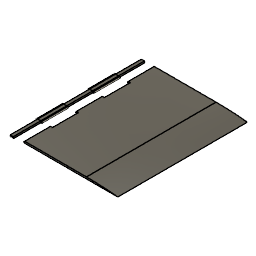
Expandable Notebook (Autodesk Fusion 360 design; units mm, degrees)
Autodesk Fusion 360 part; units mm, degrees
sketch "Sketch1" plane through (0, 0, 0) normal (0, 0, 1) x (1, 0, 0)
  line L0 (0, 0) -> (-148.5, 0)
  line L1 (-148.5, 0) -> (-148.5, 210)
  line L2 (-148.5, 210) -> (0, 210)
  line L3 (0, 210) -> (0, 0)
  line L4 (0, 0) -> (7.0711, -7.0711)
  line L5 (0, 0) -> (10, 0) construction
  line L6 (-148.5, 210) -> (-155.5711, 217.0711)
  line L7 (-148.5, 210) -> (-138.5, 210) construction
  line L8 (-155.5711, 217.0711) -> (7.0711, 217.0711)
  line L9 (7.0711, 217.0711) -> (7.0711, -7.0711)
  line L10 (7.0711, -7.0711) -> (-155.5711, -7.0711)
  line L11 (-155.5711, -7.0711) -> (-155.5711, 217.0711)
  dimension "d1" = 148.5
  dimension "d2" = 210
  dimension "d3" = 10
  dimension "d4" = 45
  dimension "d5" = 135
  dimension "d6" = 10
  constraint horizontal L0
  constraint vertical L1
  constraint horizontal L2
  constraint vertical L3
  constraint coincident L0.start L3.end
  constraint horizontal L5
  constraint horizontal L7
  constraint horizontal L8
  constraint vertical L9
  constraint horizontal L10
  constraint vertical L11
  measures "d1" distance of L0.start L0.end
  measures "d2" distance of L0.start L2.end
  measures "d3" distance of L0.start L4.end
  measures "d4" angle of L4 L5
  measures "d5" angle of L6 L7
  measures "d6" distance of L1.end L6.end
extrude "Extrude1" add sketch "Sketch1" along normal blind 3 makes body 1
sketch "Sketch2" plane through (0, 0, 3) normal (0, 0, 1) x (-1, 0, 0)
  line L0 (155.5711, 7.0711) -> (-7.0711, 7.0711)
  line L1 (-7.0711, 7.0711) -> (-7.0711, -217.0711)
  line L2 (-7.0711, -217.0711) -> (155.5711, -217.0711)
  line L3 (155.5711, -217.0711) -> (155.5711, 7.0711)
  line L4 (155.5711, 7.0711) -> (145.5711, 7.0711)
  line L5 (145.5711, 7.0711) -> (145.5711, -217.0709)
  line L6 (145.5711, -217.0709) -> (155.5711, -217.0709)
  line L7 (155.5711, -217.0709) -> (155.5711, 7.0711)
  line L8 (155.5711, -217.0711) -> (150.5711, -217.0711)
  line L9 (150.5711, -217.0711) -> (150.5711, -172.2427)
  line L10 (150.5711, -172.2427) -> (155.5711, -172.2427)
  line L11 (155.5711, -172.2427) -> (155.5711, -217.0711)
  line L12 (150.5711, -172.2427) -> (155.5711, -172.2427)
  line L13 (155.5711, -172.2427) -> (155.5711, -127.4143)
  line L14 (155.5711, -127.4143) -> (150.5711, -127.4143)
  line L15 (150.5711, -127.4143) -> (150.5711, -172.2427)
  line L16 (150.5711, -127.4143) -> (155.5711, -127.4143)
  line L17 (155.5711, -127.4143) -> (155.5711, -82.5859)
  line L18 (155.5711, -82.5859) -> (150.5711, -82.5859)
  line L19 (150.5711, -82.5859) -> (150.5711, -127.4143)
  line L20 (150.5711, -82.5859) -> (155.5711, -82.5859)
  line L21 (155.5711, -82.5859) -> (155.5711, -37.7575)
  line L22 (155.5711, -37.7575) -> (150.5711, -37.7575)
  line L23 (150.5711, -37.7575) -> (150.5711, -82.5859)
  line L24 (150.5711, -37.7575) -> (155.5711, -37.7575)
  line L25 (155.5711, -37.7575) -> (155.5711, 7.0711)
  line L26 (155.5711, 7.0711) -> (150.5711, 7.0711)
  line L27 (150.5711, 7.0711) -> (150.5711, -37.7575)
  dimension "d9" = 10
  dimension "d10" = 224.142
  dimension "d11" = 44.8284
  dimension "d12" = 44.8284
  dimension "d13" = 44.8284
  dimension "d14" = 44.8284
  constraint horizontal L4
  constraint vertical L5
  constraint horizontal L6
  constraint vertical L7
  constraint coincident L0.start L3.end
  constraint horizontal L8
  constraint vertical L9
  constraint horizontal L10
  constraint vertical L11
  constraint coincident L2.end L3.start
  constraint horizontal L12
  constraint vertical L13
  constraint horizontal L14
  constraint vertical L15
  constraint horizontal L16
  constraint vertical L17
  constraint horizontal L18
  constraint vertical L19
  constraint coincident L7 L17.end
  constraint horizontal L20
  constraint vertical L21
  constraint horizontal L22
  constraint vertical L23
  constraint coincident L7 L21.end
  constraint horizontal L24
  constraint vertical L25
  constraint horizontal L26
  constraint vertical L27
  measures "d9" distance of L0.start L4.end
  measures "d10" distance of L0.start L6.end
  measures "d11" distance of L2.end L10.end
  measures "d12" distance of L9.end L14.end
  measures "d13" distance of L14.end L18.end
  measures "d14" distance of L18.end L22.end
extrude "Extrude2" cut sketch "Sketch2" against normal blind 160 contours L3 L7 L18 L20 L21 L22 L23 L24 | L3 L7 L10 L12 L13 L14 L15 L16 bodies 1
sketch "Sketch3" plane through (0, 0, 0) normal (0, 0, 1) x (1, 0, 0)
  line L0 (-170.5711, 217.0711) -> (-176.0711, 217.0711)
  line L1 (-176.0711, 217.0711) -> (-176.0711, -9.7901)
  line L2 (-176.0711, -9.7901) -> (-170.5711, -9.7901)
  line L3 (-170.5711, -9.7901) -> (-170.5711, 217.0711)
  line L4 (-170.5711, 217.0711) -> (-170.5711, 172.2427)
  line L5 (-170.5711, 127.4143) -> (-170.5711, 82.5859)
  line L6 (-170.5711, 82.5859) -> (-170.5711, 37.7575)
  line L7 (-170.5711, 37.7575) -> (-167.5711, 37.7575)
  line L8 (-167.5711, 37.7575) -> (-167.5711, 82.5859)
  line L9 (-167.5711, 82.5859) -> (-170.5711, 82.5859)
  line L10 (-170.5711, 82.5859) -> (-170.5711, 37.7575)
  line L11 (-176.0711, 172.2427) -> (-179.0711, 172.2427)
  line L12 (-179.0711, 172.2427) -> (-179.0711, 127.4143)
  line L13 (-179.0711, 127.4143) -> (-176.0711, 127.4143)
  line L14 (-176.0711, 127.4143) -> (-176.0711, 172.2427)
  line L15 (-170.5711, 82.5859) -> (-176.0711, 82.5859)
  line L16 (-176.0711, 82.5859) -> (-176.0711, 37.7575)
  line L17 (-176.0711, 37.7575) -> (-170.5711, 37.7575)
  line L18 (-170.5711, 37.7575) -> (-170.5711, 82.5859)
  line L19 (-176.0711, 37.7575) -> (-179.0711, 37.7575)
  line L20 (-179.0711, 37.7575) -> (-179.0711, 82.5859)
  line L21 (-179.0711, 82.5859) -> (-176.0711, 82.5859)
  line L22 (-176.0711, 82.5859) -> (-176.0711, 37.7575)
  line L23 (-170.5711, 172.2427) -> (-167.5711, 172.2427)
  line L24 (-167.5711, 172.2427) -> (-167.5711, 127.4143)
  line L25 (-167.5711, 127.4143) -> (-170.5711, 127.4143)
  line L26 (-170.5711, 127.4143) -> (-170.5711, 172.2427)
  point P0 (-155.5711, 217.0711)
  point P1 (-155.5711, -7.0711)
  dimension "d17" = 15
  dimension "d19" = 5.5
  dimension "d20" = 44.8284
  dimension "d21" = 44.8284
  dimension "d22" = 44.8284
  dimension "d23" = 44.8284
  dimension "d24" = 3
  dimension "d25" = 44.8284
  dimension "d27" = 3
  dimension "d28" = 44.8284
  dimension "d29" = 3
  dimension "d30" = 3
  dimension "d31" = 44.8284
  constraint horizontal L0
  constraint vertical L1
  constraint horizontal L2
  constraint vertical L3
  constraint coincident L3 L5.start
  constraint horizontal L7
  constraint vertical L8
  constraint horizontal L9
  constraint vertical L10
  constraint horizontal L11
  constraint vertical L12
  constraint horizontal L13
  constraint vertical L14
  constraint coincident L1 L11.start
  constraint horizontal L15
  constraint vertical L16
  constraint horizontal L17
  constraint vertical L18
  constraint coincident L1 L16.end
  constraint horizontal L19
  constraint vertical L20
  constraint horizontal L21
  constraint vertical L22
  constraint horizontal L23
  constraint vertical L24
  constraint horizontal L25
  constraint vertical L26
  measures "d17" distance of P0 L0.start
  measures "d19" distance of L0.start L0.end
  measures "d20" distance of L0.start L4.end
  measures "d21" distance of L4.end L5.start
  measures "d22" distance of L5.start L5.end
  measures "d23" distance of L5.end L6.end
  measures "d24" distance of L6.end L7.end
  measures "d25" distance of L6.end L5.end
  measures "d27" distance of L11.start L11.end
  measures "d28" distance of L5.end L6.end
  measures "d29" distance of L16.end L19.end
  measures "d30" distance of L4.end L23.end
  measures "d31" distance of L4.end L5.start
extrude "Extrude3" add sketch "Sketch3" along normal blind 3 separate body makes body 2
fillet "Fillet1" radius 1.5 8 edges at (-179.0711, 60.1717, 0) (-179.0711, 60.1717, 3) (-179.0711, 149.8285, 0) (-179.0711, 149.8285, 3) (-167.5711, 60.1717, 0) (-167.5711, 60.1717, 3) (-167.5711, 149.8285, 0) (-167.5711, 149.8285, 3) on bodies 2
fillet "Fillet2" radius 1.5 6 edges at (-155.5711, 194.6569, 3) (-155.5711, 194.6569, 0) (-155.5711, 105.0001, 0) (-155.5711, 105.0001, 3) (-155.5711, 15.3432, 3) (-155.5711, 15.3432, 0) on bodies 1
sketch "Sketch4" plane through (0, 217.0711, 0) normal (0, 1, 0) x (-1, 0, 0)
  line L0 (170.5711, 0) -> (176.0711, 0)
  line L1 (176.0711, 0) -> (176.0711, 3)
  line L2 (176.0711, 3) -> (170.5711, 3)
  line L3 (170.5711, 3) -> (170.5711, 0)
  line L4 (170.5711, 3) -> (176.0711, 3)
  line L5 (173.3211, 3) -> (173.3211, 2)
  line L6 (173.3211, 2) -> (170.5711, 3)
  line L7 (173.3211, 2) -> (176.0711, 3)
  constraint coincident L2.end L3.start
  constraint coincident L1.end L2.start
  constraint midpoint L4 L5.start
  constraint perpendicular L4 L5
extrude "Extrude4" cut sketch "Sketch4" against normal blind 240 contours L2 L4 L5 L6 | L2 L4 L5 L7 bodies 2
sketch "Sketch5" plane through (0, 0, 0) normal (0, 0, -1) x (1, 0, 0)
  line L0 (-169.0711, -172.2427) -> (-169.0711, -127.4143)
  line L1 (-169.0711, -127.4143) -> (-170.5711, -127.4143)
  line L2 (-170.5711, -127.4143) -> (-170.5711, -82.5859)
  line L3 (-170.5711, -82.5859) -> (-169.0711, -82.5859)
  line L4 (-169.0711, -82.5859) -> (-169.0711, -37.7575)
  line L5 (-169.0711, -37.7575) -> (-170.5711, -37.7575)
  line L6 (-170.5711, -37.7575) -> (-170.5711, 9.7901)
  line L7 (-170.5711, 9.7901) -> (-176.0711, 9.7901)
  line L8 (-176.0711, 9.7901) -> (-176.0711, -37.7575)
  line L9 (-176.0711, -37.7575) -> (-177.5711, -37.7575)
  line L10 (-177.5711, -37.7575) -> (-177.5711, -82.5859)
  line L11 (-177.5711, -82.5859) -> (-176.0711, -82.5859)
  line L12 (-176.0711, -82.5859) -> (-176.0711, -127.4143)
  line L13 (-176.0711, -127.4143) -> (-177.5711, -127.4143)
  line L14 (-177.5711, -127.4143) -> (-177.5711, -172.2427)
  line L15 (-177.5711, -172.2427) -> (-176.0711, -172.2427)
  line L16 (-176.0711, -172.2427) -> (-176.0711, -217.0711)
  line L17 (-176.0711, -217.0711) -> (-170.5711, -217.0711)
  line L18 (-170.5711, -217.0711) -> (-170.5711, -172.2427)
  line L19 (-170.5711, -172.2427) -> (-169.0711, -172.2427)
  line L20 (-170.5711, 9.7901) -> (-176.0711, 9.7901)
  line L21 (-176.0711, 9.7901) -> (-176.0711, -217.0711)
  line L22 (-176.0711, -217.0711) -> (-170.5711, -217.0711)
  line L23 (-170.5711, -217.0711) -> (-170.5711, 9.7901)
  line L24 (-170.5711, 9.7901) -> (-173.3211, 9.7901)
  line L25 (-173.3211, 9.7901) -> (-171.9461, 9.7901)
  line L26 (-176.0711, 9.7901) -> (-173.3211, 9.7901)
  line L27 (-174.6961, 9.7901) -> (-173.3211, 9.7901)
  line L28 (-171.9461, 9.7901) -> (-173.3211, 9.7901)
  line L29 (-171.9461, 9.7901) -> (-171.9461, -217.0711)
  line L30 (-171.9461, -217.0711) -> (-174.6961, -217.0711)
  line L31 (-174.6961, -217.0711) -> (-174.6961, 9.7901)
  line L32 (-174.6961, 9.7901) -> (-171.9461, 9.7901)
  line L33 (-171.9461, 9.7901) -> (-171.9461, -217.0711)
  constraint horizontal L20
  constraint vertical L21
  constraint horizontal L22
  constraint vertical L23
  constraint coincident L16.end L17.start
  constraint coincident L6.end L7.start
  constraint midpoint L20 L24.end
  constraint midpoint L24 L25.end
  constraint coincident L7.end L8.start
  constraint midpoint L26 L27.start
  constraint coincident L22 L29.end
  constraint perpendicular L22 L29
  constraint horizontal L30
  constraint vertical L31
  constraint horizontal L32
  constraint vertical L33
extrude "Extrude5" cut sketch "Sketch5" against normal blind 1 contours L7 L17 L20 L22 L24 L25 L26 L27 L28 L29 L30 L31 L32 L33 bodies 2
fillet "Fillet3" radius 13 1 edges at (-173.3211, 103.6405, 2) on bodies 2
fillet "Fillet4" radius 0.5 2 edges at (-174.6961, 103.6405, 0) (-171.9461, 103.6405, 0) on bodies 2
sketch "Sketch6" plane through (0, 0, 1) normal (0, 0, -1) x (1, 0, 0)
  line L0 (-171.9461, 9.7901) -> (-174.6961, 9.7901)
  line L1 (-174.6961, 9.7901) -> (-174.6961, -217.0711)
  line L2 (-174.6961, -217.0711) -> (-171.9461, -217.0711)
  line L3 (-171.9461, -217.0711) -> (-171.9461, 9.7901)
  circle A0 centre (-173.3211, -207.0711) radius 0.75
  circle A1 centre (-173.3211, -197.0711) radius 0.75
  line L4 (-172.5711, -197.0711) -> (-172.5711, -207.0711)
  line L5 (-174.0711, -207.0711) -> (-174.0711, -197.0711)
  circle A2 centre (-173.3211, -10.2099) radius 0.75
  circle A3 centre (-173.3211, -0.2099) radius 0.75
  line L6 (-174.0711, -0.2099) -> (-174.0711, -10.2099)
  line L7 (-172.5711, -10.2099) -> (-172.5711, -0.2099)
  dimension "d47" = 10
  dimension "d49" = 10
  dimension "d50" = 1.5
  dimension "d51" = 1.5
  dimension "d52" = 1.5
  dimension "d53" = 1.5
  constraint coincident A1 L4.start
  constraint coincident A0 L4.end
  constraint tangent A0 L4
  constraint coincident A0 L5.start
  constraint coincident A1 L5.end
  constraint tangent A1 L5
  constraint parallel L1 L5
  constraint coincident A3 L6.start
  constraint coincident A2 L6.end
  constraint tangent A2 L6
  constraint coincident A2 L7.start
  constraint coincident A3 L7.end
  constraint tangent A3 L7
  measures "d47" distance of A2.centre A3.centre
  measures "d49" distance of A0.centre A1.centre
  measures "d50" diameter of A0
  measures "d51" diameter of A1
  measures "d52" diameter of A2
  measures "d53" diameter of A3
extrude "Extrude6" add sketch "Sketch6" along normal blind 1 draft 15 contours A0 | A0 A1 L4 L5 | A1 | A2 | A2 A3 L6 L7 | A3 bodies 2
sketch "Sketch7" plane through (0, 37.7575, 0) normal (0, -1, 0) x (1, 0, 0)
  arc A0 (-169.0711, 0) -> (-169.0711, 3) centre (-169.0711, 1.5) ccw
  line L0 (-169.0711, 3) -> (-170.5711, 3)
  line L1 (-170.5711, 3) -> (-170.5711, 0)
  line L2 (-170.5711, 0) -> (-169.0711, 0)
  circle A1 centre (-169.0711, 1.5) radius 0.9
  dimension "d56" = 1.8
  constraint concentric A0 A1
  measures "d56" diameter of A1
extrude "Extrude7" cut sketch "Sketch7" against normal blind 245 contours A1 bodies 2
sketch "Sketch8" plane through (0, -7.0711, 0) normal (0, -1, 0) x (1, 0, 0)
  arc A0 (-154.0711, 3) -> (-154.0711, 0) centre (-154.0711, 1.5) ccw
  line L0 (-154.0711, 0) -> (7.0711, 0)
  line L1 (7.0711, 0) -> (7.0711, 3)
  line L2 (7.0711, 3) -> (-154.0711, 3)
  circle A1 centre (-154.0711, 1.5) radius 0.9
  dimension "d59" = 1.8
  constraint concentric A0 A1
  measures "d59" diameter of A1
extrude "Extrude8" cut sketch "Sketch8" against normal blind 280 contours A1 bodies 1
fillet "Fillet5" radius 492.5 1 edges at (7.0711, 105, 3) on bodies 1
